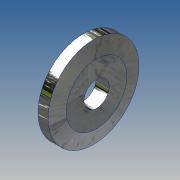
# Autodesk Inventor part: Propellerscheib_ra8846s
Saved by Autodesk Inventor 2021 (Build 250183000, 183)
## iProperties
Created: 2020-11-18
Part Number: Propellerscheib_ra8846s
Material: Aluminium 6061
Document SubType Name: Modeling
Designer: Ricardo A
Density: 2.7 g/cm^3
Appearance: Aluminium - flach
Description: Motor_Teil5_propel
Mass: 1.52639 g
Surface Area: 6.26406 cm^2
Volume: 0.56533 cm^3
Author: Sander
Autodesk Inventor part; units mm, degrees
ref_plane "YZ-Ebene" through (0, 0, 0) normal (1, 0, 0) x (0, 1, 0)
ref_plane "XZ-Ebene" through (0, 0, 0) normal (0, 1, 0) x (-1, 0, 0)
ref_plane "XY-Ebene" through (0, 0, 0) normal (0, 0, 1) x (1, 0, 0)
sketch "Skizze1" plane through (0, 0, 0) normal (0, 0, 1) x (1, 0, 0)
  line L0 (-0.52, 0) -> (3.12, 0) projected
  line L1 (0, -1.8) -> (0, 10.8) projected
  line L2 (0, 2.5) -> (2.6, 2.5)
  line L3 (2.6, 2.5) -> (2.6, 6)
  line L4 (2.6, 6) -> (2, 9)
  line L5 (2, 9) -> (0, 9)
  point P0 (0, 0)
  dimension "d0" = 2.6
  dimension "d3" = 3
  dimension "d4" = 2
  dimension "d5" = 9
  dimension "d7" = 5
  constraints: 8 end point, 2 perpendicular, 2 point on line, 1 horizontal
  measures "d0" distance of L2.start L2.end
  measures "d3" vertical distance of L3.end L4.end
  measures "d4" distance of L4.end L5.end
  measures "d5" distance from line of L0 L5.end
  measures "d7" diameter of L2.end L0
revolve "Umdrehung1" add sketch "Skizze1" angle 360 about axis through (-10, 0, 0) along (1, 0, 0)
